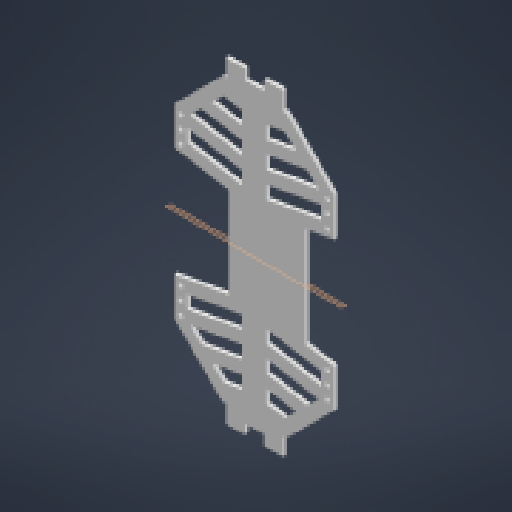
# Autodesk Inventor part: Backplane
Saved by Autodesk Inventor 2023.4 (Build 274418000, 418)
## iProperties
Created: 2025-10-02
Part Number: Backplane
Material: Generic
Document SubType Name: Modeling
Designer: Malthe Sennels
Density: 1 g/cm^3
Appearance: Default
Author: Malthe Sennels
Autodesk Inventor part; units mm, degrees
ref_plane "YZ Plane" through (0, 0, 0) normal (1, 0, 0) x (0, 1, 0)
ref_plane "XZ Plane" through (0, 0, 0) normal (0, 1, 0) x (-1, 0, 0)
ref_plane "XY Plane" through (0, 0, 0) normal (0, 0, 1) x (1, 0, 0)
sketch "Sketch1" plane through (0, 0, 0) normal (0, 0, 1) x (1, 0, 0)
  line L0 (0, -13.8137) -> (15, -13.8137) projected
  line L1 (0, 0) -> (0, -13.8137) projected
  line L2 (45, 0) -> (0, 0) projected
  line L3 (45, 0) -> (45, -13.8137) projected
  line L4 (30, -13.8137) -> (45, -13.8137) projected
  line L5 (30, -6) -> (30, -13.8137) projected
  line L6 (30, -6) -> (15, -6) projected
  line L7 (15, -6) -> (15, -13.8137) projected
  line L8 (-2.5, 0) -> (-2.5, -11.3137) projected
  line L9 (47.5, 0) -> (-2.5, 0) projected
  line L10 (47.5, 0) -> (85, 37.5)
  line L11 (47.5, 0) -> (100.533, 0) construction
  line L12 (85, 37.5) -> (85, 67.5)
  line L13 (85, 67.5) -> (62.5, 71.4674)
  line L14 (62.5, 71.4674) -> (62.5, 110.5752)
  line L15 (22.5, -6) -> (22.5, 110.5752)
  line L16 (-10.9317, 221.1504) -> (1.7683, 221.1504) construction
  line L17 (22.5, 0) -> (22.5, 221.1504)
  line L18 (22.5, 110.5752) -> (62.5, 110.5752) construction
  line L19 (-2.5, 0) -> (-40, 37.5)
  line L20 (-40, 37.5) -> (-40, 67.5)
  line L21 (-40, 67.5) -> (-17.5, 71.4674)
  line L22 (-17.5, 71.4674) -> (2.5, 74.9939)
  line L23 (2.5, 74.9939) -> (2.5, 110.5752)
  line L24 (22.5, 110.5752) -> (2.5, 110.5752) construction
  line L25 (47.5, 221.1504) -> (85, 183.6504)
  line L26 (85, 183.6504) -> (85, 153.6504)
  line L27 (85, 153.6504) -> (62.5, 149.6831)
  line L28 (62.5, 149.6831) -> (62.5, 110.5752)
  line L29 (-40, 153.6504) -> (-17.5, 149.6831)
  line L30 (-40, 183.6504) -> (-40, 153.6504)
  line L31 (-2.5, 221.1504) -> (-40, 183.6504)
  line L32 (-17.5, 149.6831) -> (2.5, 146.1565)
  line L33 (2.5, 146.1565) -> (2.5, 110.5752)
  line L34 (0, 234.9641) -> (15, 234.9641)
  line L35 (0, 221.1504) -> (0, 234.9641)
  line L36 (45, 221.1504) -> (45, 234.9641)
  line L37 (30, 234.9641) -> (45, 234.9641)
  line L38 (30, 227.1504) -> (30, 234.9641)
  line L39 (30, 227.1504) -> (15, 227.1504)
  line L40 (15, 227.1504) -> (15, 234.9641)
  line L41 (47.5, 221.1504) -> (-2.5, 221.1504)
  dimension "d0" = 45
  dimension "d1" = 100
  dimension "d2" = 40
  dimension "d3" = 30
  dimension "d4" = 40
  dimension "d5" = 20
  constraints: 62 end point, 20 symmetric about line, 4 vertical, 3 horizontal, 3 midpoint, 2 point on line, 1 collinear, 1 equal length, 1 parallel, 1 perpendicular
  measures "d0" angle of L11 L10
  measures "d1" angle of L13 L12
  measures "d2" distance between parallel lines of L15 L14
  measures "d3" distance of L10.end L12.end
  measures "d4" horizontal distance of L2.start L10.end
  measures "d5" distance between parallel lines of L23 L15
extrude "Extrusion1" add sketch "Sketch1" along normal blind 3
sketch "Sketch2" plane through (0, 0, 3) normal (0, 0, 1) x (1, 0, 0)
  line L0 (45, -13.8137) -> (45, 0) projected
  line L1 (45, 0) -> (47.5, 0) projected
  line L2 (47.5, 0) -> (85, 37.5) projected
  line L3 (85, 37.5) -> (85, 67.5) projected
  line L4 (85, 67.5) -> (62.5, 71.4674) projected
  line L5 (62.5, 71.4674) -> (62.5, 149.6831) projected
  line L6 (62.5, 149.6831) -> (85, 153.6504) projected
  line L7 (85, 153.6504) -> (85, 183.6504) projected
  line L8 (85, 183.6504) -> (47.5, 221.1504) projected
  line L9 (47.5, 221.1504) -> (45, 221.1504) projected
  line L10 (45, 221.1504) -> (45, 234.9641) projected
  line L11 (45, 234.9641) -> (30, 234.9641) projected
  line L12 (30, 234.9641) -> (30, 227.1504) projected
  line L13 (30, 227.1504) -> (15, 227.1504) projected
  line L14 (15, 227.1504) -> (15, 234.9641) projected
  line L15 (15, 234.9641) -> (0, 234.9641) projected
  line L16 (0, 234.9641) -> (0, 221.1504) projected
  line L17 (0, 221.1504) -> (-2.5, 221.1504) projected
  line L18 (-2.5, 221.1504) -> (-40, 183.6504) projected
  line L19 (-40, 183.6504) -> (-40, 153.6504) projected
  line L20 (-40, 153.6504) -> (2.5, 146.1565) projected
  line L21 (2.5, 146.1565) -> (2.5, 74.9939) projected
  line L22 (2.5, 74.9939) -> (-40, 67.5) projected
  line L23 (-40, 67.5) -> (-40, 37.5) projected
  line L24 (-40, 37.5) -> (-2.5, 0) projected
  line L25 (-2.5, 0) -> (0, 0) projected
  line L26 (0, 0) -> (0, -13.8137) projected
  line L27 (0, -13.8137) -> (15, -13.8137) projected
  line L28 (15, -13.8137) -> (15, -6) projected
  line L29 (15, -6) -> (30, -6) projected
  line L30 (30, -6) -> (30, -13.8137) projected
  line L31 (30, -13.8137) -> (45, -13.8137) projected
  line L32 (-30, 41.6421) -> (-30, 59.109)
  line L33 (-30, 59.109) -> (12.5, 66.6029)
  line L34 (12.5, 66.6029) -> (12.5, 154.5475)
  line L35 (12.5, 154.5475) -> (-30, 162.0414)
  line L36 (-30, 162.0414) -> (-30, 179.5083)
  line L37 (-30, 179.5083) -> (1.6421, 211.1504)
  line L38 (1.6421, 211.1504) -> (10, 211.1504)
  line L39 (10, 211.1504) -> (10, 217.1504)
  line L40 (10, 217.1504) -> (35, 217.1504)
  line L41 (35, 217.1504) -> (35, 211.1504)
  line L42 (35, 211.1504) -> (43.3579, 211.1504)
  line L43 (43.3579, 211.1504) -> (75, 179.5083)
  line L44 (75, 179.5083) -> (75, 162.0414)
  line L45 (75, 162.0414) -> (52.5, 158.0741)
  line L46 (52.5, 158.0741) -> (52.5, 63.0764)
  line L47 (52.5, 63.0764) -> (75, 59.109)
  line L48 (75, 59.109) -> (75, 41.6421)
  line L49 (75, 41.6421) -> (43.3579, 10)
  line L50 (43.3579, 10) -> (35, 10)
  line L51 (35, 10) -> (35, 4)
  line L52 (35, 4) -> (10, 4)
  line L53 (10, 4) -> (10, 10)
  line L54 (10, 10) -> (1.6421, 10)
  line L55 (1.6421, 10) -> (-30, 41.6421)
  line L56 (12.5, 66.6029) -> (12.5, 10)
  line L57 (12.5, 10) -> (10, 10)
  line L58 (22.5, 4) -> (22.5, 217.1504) construction
  line L59 (32.5, 66.6029) -> (32.5, 10)
  line L60 (32.5, 10) -> (35, 10)
  line L61 (32.5, 66.6029) -> (32.5, 211.1504)
  line L62 (32.5, 211.1504) -> (35, 211.1504)
  line L63 (12.5, 154.5475) -> (12.5, 211.1504)
  line L64 (12.5, 211.1504) -> (10, 211.1504)
  line L65 (-30, 48.9547) -> (12.5, 56.4486)
  line L66 (-27.5843, 39.2264) -> (12.5, 46.2944)
  line L67 (-18.9521, 30.5942) -> (12.5, 36.1401)
  line L68 (-10.3199, 21.9621) -> (12.5, 25.9858)
  line L69 (-1.6878, 13.3299) -> (12.5, 15.8316)
  line L70 (75, 48.9547) -> (32.5, 56.4486)
  line L71 (72.5843, 39.2264) -> (32.5, 46.2944)
  line L72 (63.9521, 30.5942) -> (32.5, 36.1401)
  line L73 (55.3199, 21.9621) -> (32.5, 25.9858)
  line L74 (46.6878, 13.3299) -> (32.5, 15.8316)
  line L75 (52.5, 63.0764) -> (32.5, 66.6029)
  point P0 (32.5, 56.4486)
  point P1 (32.5, 46.2944)
  dimension "d8" = 10
  dimension "d9" = 10
  dimension "d10" = 10
  dimension "d11" = 10
  dimension "d12" = 10
  dimension "d13" = 10
  constraints: 88 end point, 12 symmetric about line, 10 point on line, 5 parallel, 4 perpendicular, 2 midpoint, 2 vertical, 23 other
  measures "d8" distance between parallel lines of L23 L32
  measures "d9" distance between parallel lines of L65 L33
  measures "d10" distance between parallel lines of L65 L66
  measures "d11" distance between parallel lines of L66 L67
  measures "d12" distance between parallel lines of L67 L68
  measures "d13" distance between parallel lines of L68 L69
extrude "Extrusion2" cut sketch "Sketch2" against normal blind 3 contours L32 L33 L56 L65 | L66 L56 L67 L55 | L68 L56 L69 L55 | L75 L47 L48 L70 L59 | L74 L59 L73 L49 | L71 L49 L72 L59
ref_plane "Work Plane1" through (0, 110.5752, 0) normal (0, 1, 0) x (1, 0, 0)
mirror "Mirror1" about plane through (0, 110.5752, 0) normal (0, 1, 0) of "Extrusion2"
sketch "Sketch3" plane through (0, 0, 0) normal (0, 0, -1) x (-1, 0, 0)
  line L0 (10.3199, 199.1884) -> (-12.5, 195.1646) projected
  line L1 (-12.5, 195.1646) -> (-12.5, 205.3189) projected
  line L2 (-12.5, 205.3189) -> (1.6878, 207.8205) projected
  line L3 (1.6878, 207.8205) -> (10.3199, 199.1884) projected
  line L4 (-32.5, 164.7018) -> (-32.5, 154.5475) projected
  line L5 (-32.5, 154.5475) -> (-75, 162.0414) projected
  line L6 (-75, 162.0414) -> (-75, 172.1957) projected
  line L7 (-75, 172.1957) -> (-32.5, 164.7018) projected
  line L8 (27.5843, 181.924) -> (-12.5, 174.8561) projected
  line L9 (-12.5, 174.8561) -> (-12.5, 185.0103) projected
  line L10 (-12.5, 185.0103) -> (18.9521, 190.5562) projected
  line L11 (18.9521, 190.5562) -> (27.5843, 181.924) projected
  line L12 (-46.6878, 207.8205) -> (-32.5, 205.3189) projected
  line L13 (-32.5, 205.3189) -> (-32.5, 195.1646) projected
  line L14 (-32.5, 195.1646) -> (-55.3199, 199.1884) projected
  line L15 (-55.3199, 199.1884) -> (-46.6878, 207.8205) projected
  line L16 (-63.9521, 190.5562) -> (-32.5, 185.0103) projected
  line L17 (-32.5, 185.0103) -> (-32.5, 174.8561) projected
  line L18 (-32.5, 174.8561) -> (-72.5843, 181.924) projected
  line L19 (-72.5843, 181.924) -> (-63.9521, 190.5562) projected
  line L20 (-12.5, 164.7018) -> (30, 172.1957) projected
  line L21 (30, 172.1957) -> (30, 162.0414) projected
  line L22 (30, 162.0414) -> (-12.5, 154.5475) projected
  line L23 (-12.5, 154.5475) -> (-12.5, 164.7018) projected
  line L24 (-12.5, 25.9858) -> (10.3199, 21.9621) projected
  line L25 (10.3199, 21.9621) -> (1.6878, 13.3299) projected
  line L26 (1.6878, 13.3299) -> (-12.5, 15.8316) projected
  line L27 (-12.5, 15.8316) -> (-12.5, 25.9858) projected
  line L28 (-32.5, 66.6029) -> (-32.5, 56.4486) projected
  line L29 (-32.5, 56.4486) -> (-75, 48.9547) projected
  line L30 (-75, 48.9547) -> (-75, 59.109) projected
  line L31 (-75, 59.109) -> (-32.5, 66.6029) projected
  line L32 (-12.5, 46.2944) -> (27.5843, 39.2264) projected
  line L33 (27.5843, 39.2264) -> (18.9521, 30.5942) projected
  line L34 (18.9521, 30.5942) -> (-12.5, 36.1401) projected
  line L35 (-12.5, 36.1401) -> (-12.5, 46.2944) projected
  line L36 (-32.5, 15.8316) -> (-46.6878, 13.3299) projected
  line L37 (-46.6878, 13.3299) -> (-55.3199, 21.9621) projected
  line L38 (-55.3199, 21.9621) -> (-32.5, 25.9858) projected
  line L39 (-32.5, 25.9858) -> (-32.5, 15.8316) projected
  line L40 (-32.5, 36.1401) -> (-63.9521, 30.5942) projected
  line L41 (-63.9521, 30.5942) -> (-72.5843, 39.2264) projected
  line L42 (-72.5843, 39.2264) -> (-32.5, 46.2944) projected
  line L43 (-32.5, 46.2944) -> (-32.5, 36.1401) projected
  line L44 (30, 48.9547) -> (-12.5, 56.4486) projected
  line L45 (-12.5, 56.4486) -> (-12.5, 66.6029) projected
  line L46 (-12.5, 66.6029) -> (30, 59.109) projected
  line L47 (30, 59.109) -> (30, 48.9547) projected
  line L48 (-45, -13.8137) -> (-45, 0) projected
  line L49 (-30, -13.8137) -> (-45, -13.8137) projected
  line L50 (-30, -6) -> (-30, -13.8137) projected
  line L51 (-15, -6) -> (-30, -6) projected
  line L52 (-15, -13.8137) -> (-15, -6) projected
  line L53 (0, -13.8137) -> (-15, -13.8137) projected
  line L54 (0, 0) -> (0, -13.8137) projected
  line L55 (2.5, 0) -> (0, 0) projected
  line L56 (40, 37.5) -> (2.5, 0) projected
  line L57 (40, 67.5) -> (40, 37.5) projected
  line L58 (-2.5, 74.9939) -> (40, 67.5) projected
  line L59 (-2.5, 146.1565) -> (-2.5, 74.9939) projected
  line L60 (40, 153.6504) -> (-2.5, 146.1565) projected
  line L61 (40, 183.6504) -> (40, 153.6504) projected
  line L62 (2.5, 221.1504) -> (40, 183.6504) projected
  line L63 (0, 221.1504) -> (2.5, 221.1504) projected
  line L64 (0, 234.9641) -> (0, 221.1504) projected
  line L65 (-15, 234.9641) -> (0, 234.9641) projected
  line L66 (-15, 227.1504) -> (-15, 234.9641) projected
  line L67 (-30, 227.1504) -> (-15, 227.1504) projected
  line L68 (-30, 234.9641) -> (-30, 227.1504) projected
  line L69 (-45, 234.9641) -> (-30, 234.9641) projected
  line L70 (-45, 221.1504) -> (-45, 234.9641) projected
  line L71 (-47.5, 221.1504) -> (-45, 221.1504) projected
  line L72 (-85, 183.6504) -> (-47.5, 221.1504) projected
  line L73 (-85, 153.6504) -> (-85, 183.6504) projected
  line L74 (-62.5, 149.6831) -> (-85, 153.6504) projected
  line L75 (-62.5, 71.4674) -> (-62.5, 149.6831) projected
  line L76 (-85, 67.5) -> (-62.5, 71.4674) projected
  line L77 (-85, 37.5) -> (-85, 67.5) projected
  line L78 (-47.5, 0) -> (-85, 37.5) projected
  line L79 (-45, 0) -> (-47.5, 0) projected
  circle A0 centre (35, 62.5) radius 1.75
  circle A1 centre (35, 52.5) radius 1.75
  circle A2 centre (35, 42.5) radius 1.75
  line L80 (-2.5, 146.1565) -> (-2.5, 74.9939) projected
  line L81 (-2.5, 110.5752) -> (-62.5, 110.5752)
  circle A3 centre (35, 158.6504) radius 1.75
  circle A4 centre (35, 168.6504) radius 1.75
  circle A5 centre (35, 178.6504) radius 1.75
  line L82 (-15, -6) -> (-30, -6) projected
  line L83 (-22.5, -6) -> (-22.5, 227.1504)
  line L84 (-30, 227.1504) -> (-15, 227.1504) projected
  circle A6 centre (-80, 62.5) radius 1.75
  circle A7 centre (-80, 52.5) radius 1.75
  circle A8 centre (-80, 42.5) radius 1.75
  circle A9 centre (-80, 158.6504) radius 1.75
  circle A10 centre (-80, 168.6504) radius 1.75
  circle A11 centre (-80, 178.6504) radius 1.75
  dimension "d16" = 3.5
  dimension "d19" = 10
  dimension "d24" = 5
  dimension "d25" = 5
  constraints: 12 centre point, 9 symmetric about line, 4 end point, 4 midpoint, 1 vertical, 13 other
  measures "d16" diameter of A0
  measures "d19" distance of A0.centre A1.centre
  measures "d24" distance from line of L57 A0.centre
  measures "d25" horizontal distance of L57.start A0.centre
extrude "Extrusion3" cut sketch "Sketch3" against normal through all contours A0 | A1 | A2 | A3 | A4 | A5 | A6 | A7 | A8 | A9 | A10 | A11
body "Solid1"
